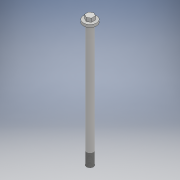
# Autodesk Inventor part: 後輪シャフト
Saved by Autodesk Inventor 2018 (Build 220112000, 112)
## iProperties
Created: 2017-09-10
Part Number: 後輪シャフト
Material: 一般
Document SubType Name: Modeling
Designer: mura5
Density: 1 g/cm^3
Appearance: 既定
Author: mura5
Autodesk Inventor part; units mm, degrees
ref_plane "YZ Plane" through (0, 0, 0) normal (1, 0, 0) x (0, 1, 0)
ref_plane "XZ Plane" through (0, 0, 0) normal (0, 1, 0) x (-1, 0, 0)
ref_plane "XY Plane" through (0, 0, 0) normal (0, 0, 1) x (1, 0, 0)
sketch "スケッチ1" plane through (0, 0, 0) normal (0, 0, 1) x (1, 0, 0)
  circle A0 centre (0, 0) radius 5.95
  dimension "d0" = 11.9
  constraints: 1 centre point, 1 coincident
  measures "d0" diameter of A0
extrude "押し出し1" add sketch "スケッチ1" along normal blind 215
thread "ねじ1" size "M12x1.75" class "6g" standard "ANSI Metric M Profile" length 22
sketch "スケッチ2" plane through (0, 0, 215) normal (0, 0, 1) x (1, 0, 0)
  circle A0 centre (0, 0) radius 11.3
  dimension "d5" = 22.6
  constraints: 1 centre point, 1 coincident
  measures "d5" diameter of A0
extrude "押し出し2" add sketch "スケッチ2" along normal blind 4.5
sketch "スケッチ3" plane through (0, 0, 219.5) normal (0, 0, 1) x (1, 0, 0)
  circle A0 centre (0, 0) radius 5.9 construction
  line L0 (5.9, -3.4064) -> (0, -6.8127)
  line L1 (0, -6.8127) -> (-5.9, -3.4064)
  line L2 (-5.9, -3.4064) -> (-5.9, 3.4064)
  line L3 (-5.9, 3.4064) -> (0, 6.8127)
  line L4 (0, 6.8127) -> (5.9, 3.4064)
  line L5 (5.9, 3.4064) -> (5.9, -3.4064)
  point P0 (5.9, 0)
  dimension "d8" = 11.8
  constraints: 12 end point, 2 coincident, 1 horizontal alignment, 1 midpoint, 15 other
extrude "押し出し3" add sketch "スケッチ3" along normal blind 6.3
